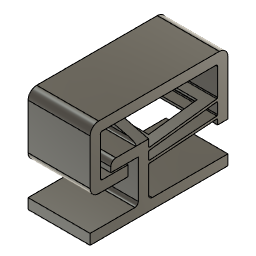
v2 (Autodesk Fusion 360 design; units mm, degrees)
Autodesk Fusion 360 part; units mm, degrees
sketch "Sketch2" plane through (0, 0, 0) normal (1, 0, 0) x (0, 1, 0)
  line L0 (0, 0) -> (40, 0)
  line L1 (40, 0) -> (40, 30)
  line L2 (40, 30) -> (0, 30)
  line L3 (0, 30) -> (0, 0)
  line L4 (3, 3) -> (37, 3)
  line L5 (37, 3) -> (37, 27)
  line L6 (37, 27) -> (3, 27)
  line L7 (3, 27) -> (3, 3)
  line L8 (17, 3) -> (17, 18.25)
  line L9 (17, 18.25) -> (6, 18.25)
  line L10 (6, 18.25) -> (6, 15.25)
  line L11 (6, 15.25) -> (14, 15.25)
  line L12 (14, 15.25) -> (14, 3)
  line L13 (3, 14.75) -> (11, 14.75)
  line L14 (11, 14.75) -> (11, 11.75)
  line L15 (11, 11.75) -> (3, 11.75)
  line L16 (3, 11.75) -> (0, 11.75)
  line L17 (37, 11.75) -> (40, 11.75)
  line L18 (17, 12) -> (37, 13.3985)
  line L19 (17, 12.7518) -> (37, 14.1504)
  line L20 (17, 15.2518) -> (37, 17.7075)
  line L21 (17, 16.0075) -> (37, 18.4632)
  line L22 (3, 3) -> (0, 3)
  line L23 (37, 3) -> (40, 3)
  dimension "d1" = -3
  dimension "d2" = 30
  dimension "d3" = 40
  dimension "d4" = 3
  dimension "d5" = 3
  dimension "d6" = 3
  dimension "d7" = 0.5
  dimension "d8" = 3
  dimension "d9" = 14
  dimension "d10" = 3
  dimension "d11" = 8.75
  dimension "d12" = 0.75
  dimension "d13" = 0.75
  dimension "d14" = 94
  dimension "d15" = 97
  dimension "d16" = 2.5
  dimension "d17" = 9
  constraint horizontal L0
  constraint vertical L1
  constraint horizontal L2
  constraint vertical L3
  constraint coincident L0.start L3.end
  constraint coincident L4 L8.start
  constraint perpendicular L4 L8
  constraint perpendicular L8 L9
  constraint perpendicular L9 L10
  constraint perpendicular L10 L11
  constraint coincident L4 L12.end
  constraint perpendicular L4 L12
  constraint perpendicular L7 L13
  constraint perpendicular L4 L14
  constraint coincident L7 L15.end
  constraint perpendicular L7 L15
  constraint coincident L3 L16.end
  constraint perpendicular L3 L16
  constraint coincident L5 L17.start
  constraint coincident L1 L17.end
  constraint perpendicular L1 L17
  constraint coincident L8 L18.start
  constraint coincident L5 L18.end
  constraint coincident L8 L19.start
  constraint coincident L5 L19.end
  constraint parallel L18 L19
  constraint coincident L8 L20.start
  constraint coincident L5 L20.end
  constraint coincident L8 L21.start
  constraint coincident L5 L21.end
  constraint parallel L20 L21
  constraint coincident L3 L22.end
  constraint perpendicular L3 L22
  constraint coincident L1 L23.end
  constraint perpendicular L1 L23
  measures "d2" distance of L0.start L2.end
  measures "d3" distance of L1.end L2.end
  measures "d4" distance of L9.end L10.end
  measures "d5" distance of L8 L12
  measures "d6" distance of L13.end L14.end
  measures "d7" distance of L11 L13
  measures "d8" distance of L12 L14
  measures "d9" distance of L3 L12
  measures "d10" distance of L7 L10
  measures "d11" distance of L6 L9
  measures "d12" distance of L18 L19
  measures "d13" distance of L20 L21
  measures "d14" angle of L8 L18
  measures "d15" angle of L8 L20
  measures "d16" distance of L19.start L20.start
  measures "d17" distance of L8.start L18.start
extrude "Extrude1" add sketch "Sketch2" along normal blind 18 contours L0 L1 L3 L4 L22 L23 | L1 L2 L3 L5 L6 L7 L16 L17 | L7 L13 L14 L15 | L4 L8 L9 L10 L11 L12 | L5 L8 L18 L19 | L5 L8 L20 L21
sketch "Sketch3" plane through (0, 0, 11.75) normal (0, 0, -1) x (1, 0, 0)
  line L0 (0, 0) -> (0, -11)
  line L1 (0, -11) -> (18, -11)
  line L2 (18, -11) -> (18, 0)
  line L3 (18, 0) -> (0, 0)
  line L4 (9, 0) -> (9, -6)
  line L5 (11.65, -8.65) -> (6.35, -8.65)
  line L6 (6.35, -8.65) -> (6.35, -3.35)
  line L7 (6.35, -3.35) -> (11.65, -3.35)
  line L8 (11.65, -3.35) -> (11.65, -8.65)
  line L9 (11.65, -8.65) -> (6.35, -3.35) construction
  line L10 (6.35, -8.65) -> (11.65, -3.35) construction
  point P0 (9, -6)
  dimension "d24" = 5.3
  dimension "d25" = 5.3
  dimension "d26" = 6
  constraint midpoint L3 L4.start
  constraint perpendicular L3 L4
  constraint horizontal L5
  constraint perpendicular L5 L6
  constraint parallel L5 L7
  constraint parallel L6 L8
  constraint coincident L9 P0
  constraint coincident L10 P0
  constraint coincident P0 L4.end
  measures "d24" distance of L6.end L7.end
  measures "d25" distance of L5.start L7.end
  measures "d26" distance of L4.start P0
extrude "Extrude2" cut sketch "Sketch3" against normal blind 5.3 contours L5 L6 L7 L8
sketch "Sketch6" plane through (0, -1.6838, 13.7134) normal (0, -0.121869, 0.992546) x (1, 0, 0)
  line L0 (0, 38.9743) -> (0, 18.8241)
  line L1 (0, 18.8241) -> (18, 18.8241)
  line L2 (18, 18.8241) -> (18, 38.9743)
  line L3 (18, 38.9743) -> (0, 38.9743)
  line L4 (0, 38.9743) -> (18, 38.9743)
  line L5 (18, 38.9743) -> (18, 18.8241)
  line L6 (18, 18.8241) -> (0, 18.8241)
  line L7 (0, 18.8241) -> (0, 38.9743)
  line L8 (3, 35.9743) -> (15, 35.9743)
  line L9 (15, 35.9743) -> (15, 21.8241)
  line L10 (15, 21.8241) -> (3, 21.8241)
  line L11 (3, 21.8241) -> (3, 35.9743)
  dimension "d34" = 3
  dimension "d35" = 3
  dimension "d36" = 3
  dimension "d37" = 3
  constraint horizontal L4
  constraint vertical L5
  constraint horizontal L6
  constraint vertical L7
  constraint coincident L1.end L2.start
  constraint coincident L0.start L3.end
  constraint horizontal L8
  constraint vertical L9
  constraint horizontal L10
  constraint vertical L11
  measures "d34" distance of L7 L11
  measures "d35" distance of L5 L9
  measures "d36" distance of L4 L8
  measures "d37" distance of L6 L10
sketch "Sketch7" plane through (0, -0.8046, 11.5068) normal (0, -0.069756, 0.997564) x (1, 0, 0)
  line L0 (0, 37.8969) -> (0, 17.8481)
  line L1 (0, 17.8481) -> (18, 17.8481)
  line L2 (18, 17.8481) -> (18, 37.8969)
  line L3 (18, 37.8969) -> (0, 37.8969)
  line L4 (0, 37.8969) -> (18, 37.8969)
  line L5 (18, 37.8969) -> (18, 17.8481)
  line L6 (18, 17.8481) -> (0, 17.8481)
  line L7 (0, 17.8481) -> (0, 37.8969)
  line L8 (3, 34.8969) -> (15, 34.8969)
  line L9 (15, 34.8969) -> (15, 20.8481)
  line L10 (15, 20.8481) -> (3, 20.8481)
  line L11 (3, 20.8481) -> (3, 34.8969)
  dimension "d38" = 3
  dimension "d39" = 3
  dimension "d40" = 3
  dimension "d41" = 3
  constraint horizontal L4
  constraint vertical L5
  constraint horizontal L6
  constraint vertical L7
  constraint coincident L1.end L2.start
  constraint coincident L0.start L3.end
  constraint horizontal L8
  constraint vertical L9
  constraint horizontal L10
  constraint vertical L11
  measures "d38" distance of L5 L9
  measures "d39" distance of L7 L11
  measures "d40" distance of L4 L8
  measures "d41" distance of L6 L10
extrude "Extrude5" cut sketch "Sketch6" against normal blind 1 contours L8 L9 L10 L11
extrude "Extrude6" cut sketch "Sketch7" against normal blind 1 contours L8 L9 L10 L11
fillet "Fillet1" radius 2.5 3 edges at (9, 0, 30) (9, 40, 30) (9, 0, 11.75)
fillet "Fillet1" radius 0.5 3 edges at (9, 3, 14.75) (9, 37, 27) (9, 3, 27)
fillet "Fillet2" radius 1 2 edges at (9, 14, 3) (9, 17, 3)
sketch "Sketch8" plane through (0, 0, 18.25) normal (0, 0, 1) x (-1, 0, 0)
  line L0 (-18, -6) -> (-18, -17)
  line L1 (-18, -17) -> (0, -17)
  line L2 (0, -17) -> (0, -6)
  line L3 (0, -17) -> (-18, -17)
  line L4 (-18, -17) -> (-18, -14)
  line L5 (-18, -14) -> (0, -14)
  line L6 (0, -14) -> (0, -17)
  line L7 (0, -6) -> (-18, -6)
  dimension "d54" = 3
  constraint horizontal L3
  constraint vertical L4
  constraint horizontal L5
  constraint vertical L6
  constraint coincident L0 L4.end
  constraint coincident L1.end L2.start
  measures "d54" distance of L1.end L5.end
extrude "Extrude7" add sketch "Sketch8" along normal blind 2 contours L0 L1 L2 L3 L4 L5 L6
chamfer "Chamfer1" distance 8 distance2 1.99 2 edges at (18, 15.5, 20.25) (0, 15.5, 20.25) measured on face at (6, 16, 20.25) measured on face at (6, 16, 20.25)
fillet "Fillet3" radius 1.5 1 edges at (9, 6, 18.25)
fillet "Fillet3" radius 0.75 1 edges at (9, 14, 18.25)
fillet "Fillet4" radius 0.25 8 edges at (9, 17, 16.0075) (9, 37, 18.4632) (9, 37, 17.7075) (9, 37, 13.3985) (9, 17, 12.7518) (9, 17, 15.2518) (9, 37, 14.1504) (9, 17, 12)
sketch "Sketch4" plane through (0, 0, 3) normal (0, 0, 1) x (-1, 0, 0)
  line L0 (0, -13) -> (0, 0)
  line L1 (0, 0) -> (-18, 0)
  line L2 (-18, 0) -> (-18, -13)
  line L3 (-3.5, -10) -> (-14.5, -10)
  line L4 (-14.5, -10) -> (-14.5, 10)
  line L5 (-14.5, 10) -> (-3.5, 10)
  line L6 (-3.5, 10) -> (-3.5, -10)
  line L7 (-3.5, -10) -> (-14.5, 10) construction
  line L8 (-14.5, -10) -> (-3.5, 10) construction
  line L9 (-14.5, -10) -> (-18, -10)
  line L10 (-18, -13) -> (0, -13)
  point P0 (-9, 0)
  dimension "d27" = 11
  dimension "d28" = 20
  constraint horizontal L3
  constraint perpendicular L3 L4
  constraint parallel L3 L5
  constraint parallel L4 L6
  constraint coincident L7 P0
  constraint coincident L8 P0
  constraint midpoint L1 P0
  constraint coincident L2 L9.end
  constraint perpendicular L2 L9
  measures "d27" distance of L3.start L3.end
  measures "d28" distance of L3.end L4.end
extrude "Extrude3" [rolled back] along distance -6 taper angle 0
sketch "Sketch5" plane through (0, 0, 3) normal (0, 0, 1) x (-1, 0, 0)
  line L0 (0, -40) -> (0, -18)
  line L1 (-18, -18) -> (-18, -40)
  line L2 (-18, -40) -> (0, -40)
  line L3 (-18, -18) -> (-4, -18)
  line L4 (-4, -18) -> (-4, -40)
  line L5 (-4, -40) -> (-18, -40)
  line L6 (-18, -40) -> (-18, -18)
  line L7 (0, -18) -> (-18, -18)
  dimension "d31" = 14
  constraint horizontal L3
  constraint vertical L4
  constraint horizontal L5
  constraint vertical L6
  constraint coincident L2 L4.end
  constraint coincident L1.start L3.start
  measures "d31" distance of L4.end L1.end
extrude "Extrude4" [rolled back] along distance -5 taper angle 0
